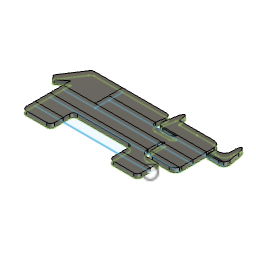
cow-as-flag (Autodesk Fusion 360 design; units mm, degrees)
Autodesk Fusion 360 part; units mm, degrees
sketch "Sketch1" plane through (0, 0, 0) normal (0, 0, 1) x (1, 0, 0)
  line L0 (162.2982, -39.1987) -> (161.1958, -32.5752)
  spline S0 degree 3 poles (161.1958, -32.5752) (160.8402, -30.4504) (160.0133, -28.7078) (159.3554, -28.7078) knots 0 0 0 0 1 1 1 1
  spline S1 degree 3 poles (159.3554, -28.7078) (158.6975, -28.7078) (158.1552, -30.4681) (158.1552, -32.6286) knots 0 0 0 0 1 1 1 1
  line L1 (158.1552, -32.6286) -> (158.1552, -34.3622)
  spline S2 degree 3 poles (158.1552, -34.3622) (158.1552, -36.5227) (156.3948, -38.283) (154.2344, -38.283) knots 0 0 0 0 1 1 1 1
  line L2 (154.2344, -38.283) -> (152.5008, -38.283)
  spline S3 degree 3 poles (152.5008, -38.283) (152.3763, -38.283) (152.2518, -38.2919) (152.1273, -38.2919) knots 0 0 0 0 1 1 1 1
  line L3 (152.1273, -38.2919) -> (152.1273, -43.0573)
  spline S4 degree 3 poles (152.1273, -43.0573) (152.2518, -43.0662) (152.3763, -43.0662) (152.5008, -43.0662) knots 0 0 0 0 1 1 1 1
  line L4 (152.5008, -43.0662) -> (159.0176, -43.0662)
  spline S5 degree 3 poles (159.0176, -43.0662) (161.178, -43.0662) (162.6538, -41.3236) (162.2982, -39.1987) knots 0 0 0 0 1 1 1 1
  line L5 (146.6774, -33.5888) -> (136.1065, -33.5888)
  spline S6 degree 3 poles (136.1065, -33.5888) (136.0176, -33.5888) (135.9287, -33.5976) (135.8486, -33.5976) knots 0 0 0 0 1 1 1 1
  line L6 (135.8486, -33.5976) -> (125.0021, -33.5976)
  spline S7 degree 3 poles (125.0021, -33.5976) (124.8776, -33.5976) (124.7532, -33.6065) (124.6287, -33.6332) knots 0 0 0 0 1 1 1 1
  line L7 (124.6287, -33.6332) -> (124.6287, -32.6286)
  spline S8 degree 3 poles (124.6287, -32.6286) (124.6287, -30.4681) (124.0864, -28.7078) (123.4284, -28.7078) knots 0 0 0 0 1 1 1 1
  spline S9 degree 3 poles (123.4284, -28.7078) (122.7705, -28.7078) (121.9437, -30.4504) (121.5881, -32.5752) knots 0 0 0 0 1 1 1 1
  line L8 (121.5881, -32.5752) -> (120.4856, -39.1987)
  spline S10 degree 3 poles (120.4856, -39.1987) (120.13, -41.3236) (121.6059, -43.0662) (123.7574, -43.0662) knots 0 0 0 0 1 1 1 1
  line L9 (123.7574, -43.0662) -> (130.2742, -43.0662)
  spline S11 degree 3 poles (130.2742, -43.0662) (130.941, -43.0662) (131.5811, -42.9595) (132.1323, -42.7817) knots 0 0 0 0 1 1 1 1
  spline S12 degree 3 poles (132.1323, -42.7817) (131.9279, -43.893) (130.9499, -44.7376) (129.7852, -44.7376) knots 0 0 0 0 1 1 1 1
  line L10 (129.7852, -44.7376) -> (120.6457, -44.7376)
  spline S13 degree 3 poles (120.6457, -44.7376) (119.1698, -44.7376) (118.0407, -43.4129) (118.2808, -41.9548) knots 0 0 0 0 1 1 1 1
  line L11 (118.2808, -41.9548) -> (119.2054, -36.3982)
  spline S14 degree 3 poles (119.2054, -36.3982) (119.4454, -34.9401) (118.3252, -33.6154) (116.8405, -33.6154) knots 0 0 0 0 1 1 1 1
  line L12 (116.8405, -33.6154) -> (71.3561, -33.6154)
  spline S15 degree 3 poles (71.3561, -33.6154) (70.387, -33.6154) (69.5513, -34.1933) (69.1779, -35.0201) knots 0 0 0 0 1 1 1 1
  line L13 (69.1779, -35.0201) -> (60.6073, -48.0538)
  spline S16 degree 3 poles (60.6073, -48.0538) (60.4651, -48.2761) (60.4829, -48.5606) (60.6518, -48.765) knots 0 0 0 0 1 1 1 1
  line L14 (60.6518, -48.765) -> (62.3143, -50.7299)
  spline S17 degree 3 poles (62.3143, -50.7299) (62.5188, -50.9788) (62.8833, -51.0144) (63.1412, -50.8099) knots 0 0 0 0 1 1 1 1
  line L15 (63.1412, -50.8099) -> (68.9645, -46.2134)
  line L16 (68.9645, -46.2134) -> (68.9645, -74.0944)
  spline S18 degree 3 poles (68.9645, -74.0944) (68.9645, -75.4191) (70.0403, -76.486) (71.3561, -76.486) knots 0 0 0 0 1 1 1 1
  line L17 (71.3561, -76.486) -> (84.2742, -76.486)
  spline S19 degree 3 poles (84.2742, -76.486) (85.5989, -76.486) (86.6658, -75.4102) (86.6658, -74.0944) knots 0 0 0 0 1 1 1 1
  line L18 (86.6658, -74.0944) -> (86.6658, -64.3947)
  spline S20 degree 3 poles (86.6658, -64.3947) (86.6658, -63.07) (87.7415, -62.0032) (89.0573, -62.0032) knots 0 0 0 0 1 1 1 1
  line L19 (89.0573, -62.0032) -> (121.2947, -62.0032)
  spline S21 degree 3 poles (121.2947, -62.0032) (122.6194, -62.0032) (123.6863, -63.0789) (123.6863, -64.3947) knots 0 0 0 0 1 1 1 1
  line L20 (123.6863, -64.3947) -> (123.6863, -74.0944)
  spline S22 degree 3 poles (123.6863, -74.0944) (123.6863, -75.4191) (124.7621, -76.486) (126.0779, -76.486) knots 0 0 0 0 1 1 1 1
  line L21 (126.0779, -76.486) -> (138.9959, -76.486)
  spline S23 degree 3 poles (138.9959, -76.486) (140.3206, -76.486) (141.3875, -75.4102) (141.3875, -74.0944) knots 0 0 0 0 1 1 1 1
  line L22 (141.3875, -74.0944) -> (141.3875, -63.6568)
  line L23 (141.3875, -63.6568) -> (134.524, -63.6568)
  spline S24 degree 3 poles (134.524, -63.6568) (132.3635, -63.6568) (130.6032, -61.8965) (130.6032, -59.7361) knots 0 0 0 0 1 1 1 1
  line L24 (130.6032, -59.7361) -> (130.6032, -53.0236)
  spline S25 degree 3 poles (130.6032, -53.0236) (130.6032, -51.7434) (131.2255, -50.6143) (132.1768, -49.8941) knots 0 0 0 0 1 1 1 1
  line L25 (132.1768, -49.8941) -> (132.1768, -57.9046)
  spline S26 degree 3 poles (132.1768, -57.9046) (132.1768, -60.065) (133.9372, -61.8254) (136.0976, -61.8254) knots 0 0 0 0 1 1 1 1
  line L26 (136.0976, -61.8254) -> (146.6685, -61.8254)
  spline S27 degree 3 poles (146.6685, -61.8254) (148.829, -61.8254) (150.5893, -60.065) (150.5893, -57.9046) knots 0 0 0 0 1 1 1 1
  line L27 (150.5893, -57.9046) -> (150.5893, -37.5095)
  spline S28 degree 3 poles (150.5893, -37.5095) (150.5982, -35.358) (148.8289, -33.5888) (146.6774, -33.5888) knots 0 0 0 0 1 1 1 1
  line L28 (89.0523, -33.6154) -> (89.0523, -50.8)
  line L29 (89.0523, -50.8) -> (68.9645, -50.8)
  line L30 (89.0523, -42.2077) -> (161.3336, -42.2077)
  line L31 (89.0523, -50.8) -> (150.5893, -50.8)
  line L32 (68.9645, -59.094) -> (150.4046, -59.094)
  line L33 (68.9645, -68.4721) -> (141.3886, -68.4721)
  line L34 (150.5893, -42.2077) -> (152.1273, -42.2077)
  line L35 (152.1273, -42.2077) -> (152.1273, -39.2757)
  line L36 (152.1273, -39.2757) -> (150.5893, -39.2757)
  line L37 (150.5893, -39.2757) -> (150.5893, -42.2077)
  constraint coincident L12 L28.start
  constraint perpendicular L12 L28
  constraint coincident L16 L29.end
  constraint perpendicular L16 L29
  constraint midpoint L28 L30.start
  constraint coincident S5 L30.end
  constraint perpendicular L3 L30
  constraint coincident L27 L31.end
  constraint perpendicular L27 L31
  constraint coincident L16 L32.start
  constraint coincident S27 L32.end
  constraint perpendicular L16 L32
  constraint horizontal L33
  constraint coincident L16 L33.start
  constraint horizontal L34
  constraint vertical L35
  constraint horizontal L36
  constraint vertical L37
  constraint coincident L3 L35.end
  constraint coincident L27 L34.start
  constraint coincident L30 L34.start
extrude "Extrude1" add sketch "Sketch1" along normal blind 2.54 contours L12 S15 L13 S16 L14 S17 L15 L16 L28 L29 makes body 1
extrude "Extrude2" add sketch "Sketch1" along normal blind 2.54 separate body contours L0 S0 S1 L1 S2 L2 S3 L3 S5 L30 L35 | L5 S6 L6 S7 L7 S8 S9 L8 S10 L27 S28 L30 L37 | S13 L11 S14 L12 L28 L30 makes body 2 at (108.0578, -39.2593, 0) makes body 3 at (135.9622, -39.3377, 0) makes body 4 at (156.2453, -40.8527, 0)
extrude "Extrude3" add sketch "Sketch1" along normal blind 2.54 separate body contours S10 L9 S11 S12 L10 S13 S25 L25 L27 L28 L30 L31 makes body 5
extrude "Extrude4" add sketch "Sketch1" along normal blind 2.54 separate body contours L25 S26 S27 L27 L31 L32 | L16 L24 S25 L29 L31 L32 makes body 6 at (89.5108, -54.3059, 0) makes body 7 at (138.3143, -53.1682, 0)
extrude "Extrude5" add sketch "Sketch1" along normal blind 2.54 separate body contours S26 L26 S27 L32 | L16 L18 S20 L19 S21 L20 L22 L23 S24 L24 L32 L33 makes body 8 at (74.8649, -63.987, 0) makes body 9 at (138.3759, -59.094, 0.8467)
extrude "Extrude6" add sketch "Sketch1" along normal blind 2.54 separate body contours L16 S18 L17 S19 L18 L33 | L20 S22 L21 S23 L22 L33 makes body 10 at (75.6621, -71.1434, 0) makes body 11 at (134.6899, -71.1434, 0)
extrude "Extrude7" add sketch "Sketch1" along normal blind 2.54 separate body contours L3 S4 L4 S5 L30 makes body 12
extrude "Extrude8" add sketch "Sketch1" along normal blind 1.27 separate body contours L3 L27 L30 L34 L35 L36 L37 makes body 13
